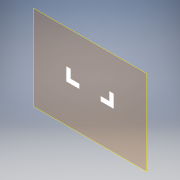
# Autodesk Inventor part: RetroTape
Saved by Autodesk Inventor 2018 (Build 220112000, 112)
## iProperties
Created: 2017-09-17
Part Number: RetroTape
Material: Generic
Document SubType Name: Modeling
Designer: Techbrick Alt
Density: 1 g/cm^3
Appearance: PTFE
Author: Techbrick Alt
Autodesk Inventor part; units mm, degrees
ref_plane "YZ Plane" through (0, 0, 0) normal (1, 0, 0) x (0, 1, 0)
ref_plane "XZ Plane" through (0, 0, 0) normal (0, 1, 0) x (-1, 0, 0)
ref_plane "XY Plane" through (0, 0, 0) normal (0, 0, 1) x (1, 0, 0)
ref_plane "Work Plane1" through (0, 0, 0) normal (0, 0, 1) x (1, 0, 0)
sketch "Sketch1" plane through (0, 0, 0) normal (0, 0, 1) x (1, 0, 0)
  line L0 (-279.4, 101.6) -> (-228.6, 101.6)
  line L1 (-228.6, 101.6) -> (-228.6, 0)
  line L2 (-228.6, 0) -> (-279.4, 0)
  line L3 (-279.4, 0) -> (-279.4, 101.6)
  line L4 (-279.4, 0) -> (-127, 0)
  line L5 (-127, 0) -> (-127, -50.8)
  line L6 (-127, -50.8) -> (-279.4, -50.8)
  line L7 (-279.4, -50.8) -> (-279.4, 0)
  line L8 (228.6, 101.6) -> (279.4, 101.6)
  line L9 (279.4, 101.6) -> (279.4, 0)
  line L10 (279.4, 0) -> (228.6, 0)
  line L11 (228.6, 0) -> (228.6, 101.6)
  line L12 (127, -50.8) -> (279.4, -50.8)
  line L13 (279.4, -50.8) -> (279.4, 0)
  line L14 (279.4, 0) -> (127, 0)
  line L15 (127, 0) -> (127, -50.8)
  line L16 (-177.8, -457.2) -> (-177.8, -381) projected
  line L17 (-177.8, -381) -> (177.8, -381) projected
  line L18 (177.8, -381) -> (177.8, -457.2) projected
  line L19 (177.8, -457.2) -> (609.6, -457.2) projected
  line L20 (609.6, -457.2) -> (609.6, 457.2) projected
  line L21 (609.6, 457.2) -> (-609.6, 457.2) projected
  line L22 (-609.6, 457.2) -> (-609.6, -457.2) projected
  line L23 (-609.6, -457.2) -> (-177.8, -457.2) projected
  line L24 (228.6, 101.6) -> (228.6, 0) projected
  line L25 (228.6, 0) -> (-228.6, 0) projected
  line L26 (-228.6, 0) -> (-228.6, 101.6) projected
  line L27 (-228.6, 101.6) -> (228.6, 101.6) projected
  point P0 (0, 0)
  dimension "d0" = 50.8
  dimension "d1" = 152.4
  constraints: 32 end point, 8 parallel, 7 collinear, 4 horizontal, 4 perpendicular, 3 equal length
  measures "d0" distance of L0.start L0.end
  measures "d1" distance of L5.end L6.end
extrude "Extrusion1" add sketch "Sketch1" along normal blind 2.54 contours L0 L1 L2 L3 | L2 L4 L5 L6 L7 | L8 L9 L10 L11 | L10 L13 L12 L15 L14
body "Solid1"
